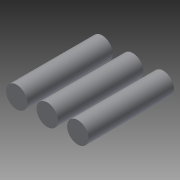
# Autodesk Inventor part: Part2
Saved by Autodesk Inventor 2014 SP1 (Build 180222100, 222)
## iProperties
Created: 2013-12-01
Part Number: Part2
Material: Generic
Document SubType Name: Modeling
Designer: Tim
Density: 1 g/cm^3
Appearance: Default
Author: Tim
Autodesk Inventor part; units mm, degrees
ref_plane "YZ Plane" through (0, 0, 0) normal (1, 0, 0) x (0, 1, 0)
ref_plane "XZ Plane" through (0, 0, 0) normal (0, 1, 0) x (-1, 0, 0)
ref_plane "XY Plane" through (0, 0, 0) normal (0, 0, 1) x (1, 0, 0)
sketch "Sketch1" plane through (0, 0, 0) normal (0, 1, 0) x (-1, 0, 0)
  circle A0 centre (-5, 0) radius 1.75
  circle A1 centre (0, 0) radius 1.75
  circle A2 centre (5, 0) radius 1.75
  dimension "d0" = 3.5
  dimension "d1" = 3.5
  dimension "d2" = 3.5
  dimension "d3" = 5
  dimension "d4" = 5
  dimension "d5" = 0
  dimension "d6" = 10
  constraints: 3 centre point
  measures "d0" diameter of A0
  measures "d1" diameter of A1
  measures "d2" diameter of A2
  measures "d3" distance of A1.centre A0.centre
  measures "d4" distance of A1.centre A2.centre
  measures "d5" distance of point (0, 0) A1.centre
  measures "d6" distance of A2.centre A0.centre
extrude "Extrusion1" add sketch "Sketch1" along normal blind 14
equation "\"d1\" = d0"
equation "\"d2\" = d0"
equation "\"d4\" = d3"
body "Solid1"
